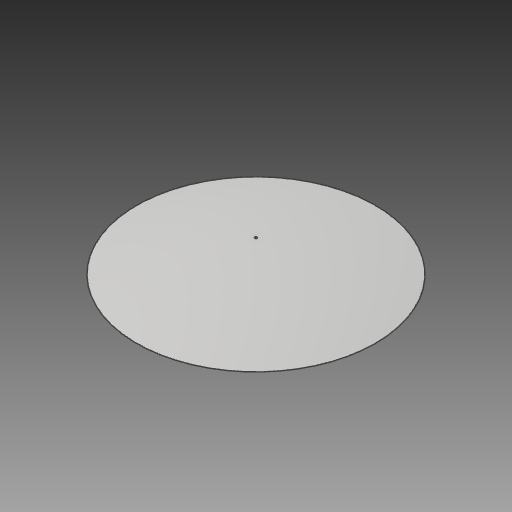
# Autodesk Inventor part: 障害物、皿
Saved by Autodesk Inventor 2017 (Build 210142000, 142)
## iProperties
Part Number: 障害物、皿
Material: 一般
Document SubType Name: Modeling
Designer: 雪村
Density: 1 g/cm^3
Appearance: 既定
Mass: 1373.44 g
Surface Area: 1462.89 cm^2
Volume: 1373.44 cm^3
Author: 雪村
Autodesk Inventor part; units mm, degrees
ref_plane "YZ Plane" through (0, 0, 0) normal (1, 0, 0) x (0, 1, 0)
ref_plane "XZ Plane" through (0, 0, 0) normal (0, 1, 0) x (-1, 0, 0)
ref_plane "XY Plane" through (0, 0, 0) normal (0, 0, 1) x (1, 0, 0)
sketch "スケッチ1" plane through (0, 0, 0) normal (0, 0, 1) x (1, 0, 0)
  line L0 (0, 0) -> (150, 0)
  line L1 (0, 0) -> (0, 40)
  arc A0 (150, 0) -> (0, 40) centre (-12.9362, -309.7609) ccw
  dimension "d0" = 150
  dimension "d1" = 40
  dimension "d2" = 350
  constraints: 4 end point, 2 point on circle, 1 centre point, 1 horizontal, 1 vertical
  measures "d0" distance of L0.start L0.end
  measures "d1" distance of L0.start L1.end
  measures "d2" radius of A0
revolve "回転1" add sketch "スケッチ1" angle 360 about axis through (0, 0, 0) along (0, -1, 0)
sketch "スケッチ2" plane through (0, 0, 0) normal (0, -1, 0) x (1, 0, 0)
  circle A0 centre (0, 0) radius 150 projected
  circle A1 centre (0, 0) radius 1.5
  dimension "d4" = 3
  constraints: 1 centre point, 1 coincident
  measures "d4" diameter of A1
extrude "押し出し1" cut sketch "スケッチ2" against normal through all contours A1
